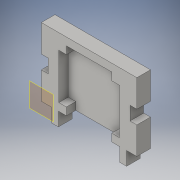
# Autodesk Inventor part: Near End Cap
Saved by Autodesk Inventor 2016 (Build 200138000, 138)
## iProperties
Created: 2016-04-25
Part Number: Near End Cap
Material: Generic
Document SubType Name: Modeling
Designer: rubenjm
Density: 1 g/cm^3
Appearance: Default
Author: rubenjm
Autodesk Inventor part; units mm, degrees
ref_plane "YZ Plane" through (0, 0, 0) normal (1, 0, 0) x (0, 1, 0)
ref_plane "XZ Plane" through (0, 0, 0) normal (0, 1, 0) x (-1, 0, 0)
ref_plane "XY Plane" through (0, 0, 0) normal (0, 0, 1) x (1, 0, 0)
sketch "Sketch1" plane through (0, 0, 0) normal (0, 0, 1) x (1, 0, 0)
  line L0 (0, 0) -> (9.525, 0)
  line L1 (88.9, 0) -> (88.9, 63.5)
  line L2 (88.9, 63.5) -> (0, 63.5)
  line L3 (0, 63.5) -> (0, 0)
  line L4 (79.375, 0) -> (79.375, -12.7)
  line L5 (79.375, -12.7) -> (73.025, -12.7)
  line L6 (73.025, -12.7) -> (73.025, 0)
  line L7 (44.45, 0) -> (44.45, 63.5) construction
  line L8 (16.25, 0) -> (16.25, 56.4) construction
  line L9 (16.25, 56.4) -> (72.65, 56.4) construction
  line L10 (72.65, 56.4) -> (72.65, 0) construction
  line L11 (9.525, 0) -> (9.525, -12.7)
  line L12 (9.525, -12.7) -> (15.875, -12.7)
  line L13 (15.875, -12.7) -> (15.875, 0)
  line L14 (15.875, 0) -> (73.025, 0)
  line L15 (79.375, 0) -> (88.9, 0)
  dimension "d0" = 88.9
  dimension "d1" = 63.5
  dimension "d4" = 6.35
  dimension "d5" = 12.7
  constraints: 32 end point, 4 parallel, 4 symmetric about line, 3 perpendicular, 1 collinear, 1 horizontal, 1 midpoint
  measures "d0" distance of L2.end L1.end
  measures "d1" distance of L1.end L1.start
  measures "d4" distance of L4.end L5.end
  measures "d5" distance of L4.start L4.end
ref_plane "Work Plane1" through (0, 0, 12.7) normal (0, 0, 1) x (1, 0, 0)
sketch "Sketch2" plane through (0, 0, 12.7) normal (0, 0, 1) x (1, 0, 0)
  line L0 (23.3366, 56.4) -> (23.3366, 49.3134)
  line L1 (65.5634, 51.3062) -> (65.5634, 49.3134)
  line L2 (23.3366, 56.4) -> (65.5634, 56.4)
  line L3 (65.5634, 56.4) -> (65.5634, 49.3134)
  line L4 (23.3366, 49.3134) -> (23.3366, 56.4)
  line L5 (65.5634, 49.3134) -> (72.65, 49.3134)
  line L6 (72.65, 49.3134) -> (72.65, 7.0866)
  line L7 (72.65, 7.0866) -> (65.5634, 7.0866)
  line L8 (23.3366, 7.0866) -> (23.3366, 0)
  line L9 (23.3366, 0) -> (65.5634, 0)
  line L10 (65.5634, 0) -> (65.5634, 7.0866)
  line L11 (23.3366, 7.0866) -> (16.25, 7.0866)
  line L12 (16.25, 7.0866) -> (16.25, 49.3134)
  line L13 (16.25, 49.3134) -> (23.3366, 49.3134)
  line L14 (44.45, 0) -> (44.45, 56.4) construction
  line L15 (28.575, 0) -> (60.325, 0) construction
  line L16 (44.45, 0) -> (44.45, 63.5) construction
  line L17 (88.9, 63.5) -> (0, 63.5) construction
  line L18 (72.65, 0) -> (16.25, 0) construction
  line L19 (16.25, 0) -> (16.25, 56.4) construction
  line L20 (16.25, 56.4) -> (72.65, 56.4) construction
  line L21 (72.65, 56.4) -> (72.65, 0) construction
  point P0 (0, 0)
  point P1 (72.65, 56.4)
  constraints: 40 end point, 6 parallel, 4 horizontal, 4 midpoint, 4 perpendicular, 2 point on line
extrude "Extrusion3" add sketch "Sketch1" along normal blind 12.7
extrude "Extrusion5" cut sketch "Sketch2" against normal blind 8.763
sketch "Sketch3" plane through (0, 0, 12.7) normal (0, 0, 1) x (1, 0, 0)
  line L0 (0, 63.5) -> (0, 0) construction
  line L1 (0, 63.5) -> (0, 0) construction
  line L2 (0, 25.4) -> (6.35, 25.4)
  line L3 (6.35, 25.4) -> (6.35, 38.1)
  line L4 (6.35, 38.1) -> (0, 38.1)
  line L5 (0, 38.1) -> (0, 25.4)
  line L6 (88.9, 63.5) -> (0, 63.5) construction
  line L7 (44.45, 63.5) -> (44.45, 0) construction
  line L8 (65.5634, 0) -> (23.3366, 0) construction
  line L9 (88.9, 25.4) -> (82.55, 25.4)
  line L10 (82.55, 25.4) -> (82.55, 38.1)
  line L11 (82.55, 38.1) -> (88.9, 38.1)
  line L12 (88.9, 38.1) -> (88.9, 25.4)
  point P0 (0, 31.75)
  point P1 (88.9, 31.75)
  dimension "d19" = 12.7
  constraints: 20 end point, 5 symmetric about line, 3 midpoint, 1 horizontal, 1 parallel, 1 perpendicular, 1 vertical
  measures "d19" distance of L3.end L2.end
extrude "Extrusion6" cut sketch "Sketch3" against normal through all
body "Solid1"
